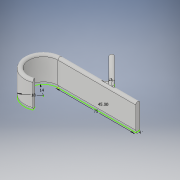
# Autodesk Inventor part: TubeRadiator
Saved by Autodesk Inventor 2019 (Build 230136000, 136)
## iProperties
Created: 2022-01-21
Part Number: TubeRadiator
Material: Generic
Document SubType Name: Modeling
Designer: talal
Density: 1 g/cm^3
Appearance: Default
Author: talal
## iProperties of the stored document TubeRadiator_3DPrint.ipt
Created: 2022-01-21
Part Number: TubeRadiator_3DPrint
Material: Generic
Document SubType Name: Modeling
Designer: talal
Density: 1 g/cm^3
Appearance: Default
Author: talal
Autodesk Inventor part; units mm, degrees
ref_plane "YZ Plane" through (0, 0, 0) normal (1, 0, 0) x (0, 1, 0)
ref_plane "XZ Plane" through (0, 0, 0) normal (0, 1, 0) x (-1, 0, 0)
ref_plane "XY Plane" through (0, 0, 0) normal (0, 0, 1) x (1, 0, 0)
sketch "Sketch1" plane through (0, 0, 0) normal (0, 1, 0) x (-1, 0, 0)
  line L0 (0, -14) -> (-75, -14)
  line L1 (-75, -14) -> (-75, -18)
  line L2 (-4.7594, 13.1662) -> (-6.5571, 16.7632)
  arc A0 (0, -14) -> (-4.7594, 13.1662) centre (0, 0) ccw
  arc A1 (0, -18) -> (-6.5571, 16.7632) centre (0, 0) ccw
  line L3 (-45, -18) -> (-21.4678, -41.5322)
  line L4 (-45, -18) -> (-11.7204, -18) construction
  line L5 (-21.4678, -41.5322) -> (-24.2962, -44.3606)
  line L6 (-24.2962, -44.3606) -> (-50.6569, -18)
  line L7 (0, -18) -> (-45, -18)
  line L8 (-50.6569, -18) -> (-75, -18)
  point P0 (0, 0)
  dimension "d3" = 75
  dimension "d4" = 14
  dimension "d5" = 18
  dimension "d6" = 45
  dimension "d7" = 4
  dimension "d8" = 4
  constraints: 18 end point, 4 point on circle, 3 horizontal, 3 perpendicular, 2 centre point, 1 collinear, 1 equal length, 1 tangent
  measures "d3" distance of L0.start L0.end
  measures "d4" radius of A0
  measures "d5" radius of A1
  measures "d6" angle of L3 L4
  measures "d7" distance of L3.end L5.end
  measures "d8" distance of L0.end L1.end
extrude "Extrusion1" add sketch "Sketch1" along normal blind 25
fillet "Fillet1" radius 2 12 edges at (-17.6881, 0, 3.3364) (22.5, 0, -18) (62.8284, 0, -18) (62.8284, 25, -18) (50.6569, 12.5, -18) (33.2339, 0, -29.7661) (37.4765, 0, -31.1803) (37.4765, 25, -31.1803) (33.2339, 25, -29.7661) (45, 12.5, -18) (-17.6881, 25, 3.3364) (22.5, 25, -18)
fillet "Fillet2" radius 2 4 edges at (37.5, 0, -14) (-13.79, 0, 2.4159) (-13.79, 25, 2.4159) (37.5, 25, -14)
sketch "Sketch2" plane through (0, 23, -14) normal (0, 0, 1) x (1, 0, 0)
  point P0 (0, -23)
sketch "Sketch3" plane through (0, 23, -14) normal (0, 0, 1) x (1, 0, 0)
  point P0 (0, -23)
sketch "Sketch4" plane through (41.5858, 2, -21.4142) normal (-0.7071, 0, 0.7071) x (0.7071, 0, 0.7071)
  line L0 (-28.4512, 21) -> (0, 21) projected
  line L1 (-17.898, 13.2543) -> (-15.2412, 14.305)
  line L2 (-15.2412, 14.305) -> (-13.0028, 12.5295)
  line L3 (-13.0028, 12.5295) -> (-13.4212, 9.7033)
  line L4 (-13.4212, 9.7033) -> (-16.078, 8.6525)
  line L5 (-16.078, 8.6525) -> (-18.3165, 10.428)
  line L6 (-18.3165, 10.428) -> (-17.898, 13.2543)
  line L7 (-12.6348, 12.4651) -> (-9.978, 13.5159)
  line L8 (-9.978, 13.5159) -> (-7.7396, 11.7404)
  line L9 (-7.7396, 11.7404) -> (-8.158, 8.9141)
  line L10 (-8.158, 8.9141) -> (-10.8148, 7.8633)
  line L11 (-10.8148, 7.8633) -> (-13.0532, 9.6388)
  line L12 (-13.0532, 9.6388) -> (-12.6348, 12.4651)
  line L13 (-15.916, 8.2429) -> (-13.2592, 9.2936)
  line L14 (-13.2592, 9.2936) -> (-11.0208, 7.5181)
  line L15 (-11.0208, 7.5181) -> (-11.4392, 4.6919)
  line L16 (-11.4392, 4.6919) -> (-14.096, 3.6411)
  line L17 (-14.096, 3.6411) -> (-16.3345, 5.4166)
  line L18 (-16.3345, 5.4166) -> (-15.916, 8.2429)
  point P0 (-14.2635, -2)
  point P1 (-12.0615, 16.231)
  constraints: 36 end point, 1 other
extrude "Extrusion2" cut sketch "Sketch4" against normal blind 1 and the other way blind 5
body "Solid1"
